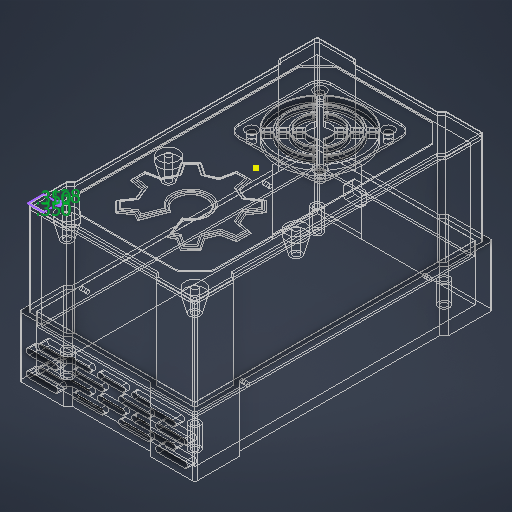
# Autodesk Inventor part: OSHE_ClassH_Enclosure_v2.0
Saved by Autodesk Inventor 2026.2 (Build 302298000, 298)
## iProperties
Created: 2026-04-01
Part Number: OSHE_ClassH_Enclosure_v2.0
Material: Generic
Document SubType Name: Modeling
Designer: ODFab
Density: 1 g/cm^3
Appearance: Default
Author: ODFab
Autodesk Inventor part; units mm, degrees
(part 1 of 2)
ref_plane "YZ Plane" through (0, 0, 0) normal (1, 0, 0) x (0, 1, 0)
ref_plane "XZ Plane" through (0, 0, 0) normal (0, 1, 0) x (-1, 0, 0)
ref_plane "XY Plane" through (0, 0, 0) normal (0, 0, 1) x (1, 0, 0)
sketch "Sketch1" plane through (0, 0, 0) normal (0, 1, 0) x (-1, 0, 0)
  line L0 (41.275, 76.2) -> (-41.275, 76.2)
  line L1 (-41.275, 76.2) -> (-41.275, -76.2)
  line L2 (-41.275, -76.2) -> (41.275, -76.2)
  line L3 (41.275, -76.2) -> (41.275, 76.2)
  line L4 (41.275, 76.2) -> (-41.275, -76.2) construction
  line L5 (-41.275, 76.2) -> (41.275, -76.2) construction
  line L6 (45.085, 80.01) -> (-45.085, 80.01)
  line L7 (-45.085, 80.01) -> (-45.085, -80.01)
  line L8 (-45.085, -80.01) -> (45.085, -80.01)
  line L9 (45.085, -80.01) -> (45.085, 80.01)
  line L10 (47.625, 82.55) -> (-47.625, 82.55)
  line L11 (-47.625, 82.55) -> (-47.625, -82.55)
  line L12 (-47.625, -82.55) -> (47.625, -82.55)
  line L13 (47.625, -82.55) -> (47.625, 82.55)
  line L14 (50.165, 85.09) -> (-50.165, 85.09)
  line L15 (-50.165, 85.09) -> (-50.165, -85.09)
  line L16 (-50.165, -85.09) -> (50.165, -85.09)
  line L17 (50.165, -85.09) -> (50.165, 85.09)
  line L18 (50.165, -85.09) -> (24.765, -85.09)
  line L19 (24.765, -85.09) -> (24.765, -59.69)
  line L20 (24.765, -59.69) -> (50.165, -59.69)
  line L21 (50.165, -59.69) -> (50.165, -85.09)
  line L22 (50.165, -59.69) -> (47.625, -59.69)
  line L23 (47.625, -59.69) -> (47.625, -57.15)
  line L24 (47.625, -57.15) -> (50.165, -57.15)
  line L25 (50.165, -57.15) -> (50.165, -59.69)
  line L26 (24.765, -82.55) -> (22.225, -82.55)
  line L27 (22.225, -82.55) -> (22.225, -85.09)
  line L28 (22.225, -85.09) -> (24.765, -85.09)
  line L29 (24.765, -85.09) -> (24.765, -82.55)
  line L30 (24.765, -85.09) -> (22.225, -82.55)
  line L31 (50.165, -59.69) -> (47.625, -57.15)
  line L32 (0, -85.09) -> (0, -83.82)
  line L33 (-50.165, 0) -> (-49.2125, 0)
  line L34 (-24.765, -85.09) -> (-22.225, -82.55)
  line L35 (-50.165, -59.69) -> (-47.625, -57.15)
  line L36 (24.765, 85.09) -> (22.225, 82.55)
  line L37 (50.165, 59.69) -> (47.625, 57.15)
  line L38 (-24.765, 85.09) -> (-22.225, 82.55)
  line L39 (-50.165, 59.69) -> (-47.625, 57.15)
  point P0 (0, 0)
  dimension "d0" = 82.55
  dimension "d1" = 152.4
  dimension "d2" = 3.81
  dimension "d3" = 2.54
  dimension "d4" = 2.54
  dimension "d5" = 25.4
  dimension "d6" = 25.4
  dimension "d7" = 2.54
  dimension "d8" = 2.54
  dimension "d9" = 2.54
  dimension "d10" = 2.54
  constraints: 80 end point, 14 parallel, 12 symmetric about line, 7 perpendicular, 5 horizontal, 4 midpoint, 2 point on line, 1 vertical, 9 other
  measures "d0" distance of L2.end L1.end
  measures "d1" distance of L1.end L0.end
  measures "d2" distance between parallel lines of L3 L9
  measures "d3" distance between parallel lines of L9 L13
  measures "d4" distance between parallel lines of L13 L17
  measures "d5" distance of L19.end L20.end
  measures "d6" distance of L18.end L19.end
  measures "d7" distance of L23.end L24.end
  measures "d8" distance of L22.end L23.end
  measures "d9" distance of L28.end L27.end
  measures "d10" distance of L27.end L26.end
extrude "Extrusion1" add sketch "Sketch1" along normal blind 31.75 contours L20 L13 L12 L19 L8 L9 | L9 L6 L7 L8 L19 L12 L11 L10 L13 L20 | L20 L17 L16 L19 L12 L13 | L13 L31 L20 | L19 L30 L12 | L13 L10 L36 L14 L17 L37 | L34 L16 L15 L35 L11 L12 | L10 L11 L39 L15 L14 L38
ref_plane "Work Plane1" through (-50.165, 0, 59.69) normal (-1, 0, 0) x (0, 0, 1)
sketch "Sketch2" plane through (-50.165, 0, 59.69) normal (-1, 0, 0) x (0, 0, 1)
  line L0 (-144.78, 0) -> (-119.38, 0) projected
  line L1 (-119.38, 0) -> (-119.38, 31.75) projected
  line L2 (-144.78, 31.75) -> (-119.38, 31.75) projected
  line L3 (-144.78, 0) -> (-144.78, 31.75) projected
  line L4 (0, 0) -> (25.4, 0) projected
  line L5 (25.4, 0) -> (25.4, 31.75) projected
  line L6 (0, 31.75) -> (25.4, 31.75) projected
  line L7 (0, 0) -> (0, 31.75) projected
  line L8 (-144.78, 31.75) -> (25.4, 31.75)
  line L9 (25.4, 31.75) -> (25.4, 0)
  line L10 (25.4, 0) -> (-144.78, 0)
  line L11 (-144.78, 0) -> (-144.78, 31.75)
  line L12 (-144.78, 0) -> (25.4, 0)
  line L13 (25.4, 0) -> (25.4, -2.54)
  line L14 (25.4, -2.54) -> (-144.78, -2.54)
  line L15 (-144.78, -2.54) -> (-144.78, 0)
  point P0 (-59.69, 0)
  point P1 (-119.38, 0)
  dimension "d14" = 2.54
  constraints: 16 end point, 4 parallel, 2 horizontal, 2 perpendicular, 1 point on line
  measures "d14" distance of L12.end L13.end
extrude "Extrusion2" add sketch "Sketch2" against normal up to surface (100.33 mm away) contours L0 L10 L4 L13 L14 L15
sketch "Sketch3" plane through (0, 31.75, 0) normal (0, 1, 0) x (1, 0, 0)
  line L0 (-47.625, 57.15) -> (-47.625, -57.15) projected
  line L1 (-47.625, -57.15) -> (-50.165, -59.69) projected
  line L2 (-50.165, -59.69) -> (-50.165, -85.09) projected
  line L3 (-50.165, -85.09) -> (-24.765, -85.09) projected
  line L4 (-24.765, -85.09) -> (-22.225, -82.55) projected
  line L5 (-22.225, -82.55) -> (22.225, -82.55) projected
  line L6 (22.225, -82.55) -> (24.765, -85.09) projected
  line L7 (24.765, -85.09) -> (50.165, -85.09) projected
  line L8 (50.165, -85.09) -> (50.165, -59.69) projected
  line L9 (50.165, -59.69) -> (47.625, -57.15) projected
  line L10 (47.625, -57.15) -> (47.625, 57.15) projected
  line L11 (47.625, 57.15) -> (50.165, 59.69) projected
  line L12 (50.165, 59.69) -> (50.165, 85.09) projected
  line L13 (50.165, 85.09) -> (24.765, 85.09) projected
  line L14 (24.765, 85.09) -> (22.225, 82.55) projected
  line L15 (22.225, 82.55) -> (-22.225, 82.55) projected
  line L16 (-22.225, 82.55) -> (-24.765, 85.09) projected
  line L17 (-24.765, 85.09) -> (-50.165, 85.09) projected
  line L18 (-50.165, 85.09) -> (-50.165, 59.69) projected
  line L19 (-50.165, 59.69) -> (-47.625, 57.15) projected
  line L20 (-45.085, 80.01) -> (45.085, 80.01) projected
  line L21 (45.085, 80.01) -> (45.085, -80.01) projected
  line L22 (45.085, -80.01) -> (-45.085, -80.01) projected
  line L23 (-45.085, -80.01) -> (-45.085, 80.01) projected
  line L24 (-50.165, 85.09) -> (50.165, 85.09)
  line L25 (50.165, 85.09) -> (50.165, -85.09)
  line L26 (50.165, -85.09) -> (-50.165, -85.09)
  line L27 (-50.165, -85.09) -> (-50.165, 85.09)
  point P0 (0, 0)
  constraints: 8 end point, 2 parallel, 1 horizontal, 1 perpendicular
extrude "Extrusion3" cut sketch "Sketch3" against normal up to surface (34.29 mm away) contours L0 L1 L27 L19 | L24 L14 L15 L16 | L4 L5 L6 L26 | L25 L9 L10 L11
sketch "Sketch4" plane through (-45.085, 0, 80.01) normal (0, 1, 0) x (1, 0, 0)
  line L0 (86.36, 3.81) -> (3.81, 3.81)
  line L1 (3.81, 3.81) -> (3.81, 156.21)
  line L2 (3.81, 156.21) -> (86.36, 156.21)
  line L3 (86.36, 156.21) -> (86.36, 3.81)
  line L4 (86.36, 3.81) -> (3.81, 156.21) construction
  line L5 (3.81, 3.81) -> (86.36, 156.21) construction
  line L6 (3.81, 156.21) -> (8.89, 156.21)
  line L7 (8.89, 156.21) -> (8.89, 151.13)
  line L8 (8.89, 151.13) -> (3.81, 151.13)
  line L9 (3.81, 151.13) -> (3.81, 156.21)
  circle A0 centre (8.89, 151.13) radius 1.7526
  line L10 (45.085, 156.21) -> (45.085, 155.0838)
  line L11 (86.36, 80.01) -> (84.9425, 80.01)
  circle A1 centre (8.89, 151.13) radius 3.0226
  circle A2 centre (81.28, 151.13) radius 1.7526
  circle A3 centre (81.28, 151.13) radius 3.0226
  circle A4 centre (8.89, 8.89) radius 1.7526
  circle A5 centre (8.89, 8.89) radius 3.0226
  circle A6 centre (81.28, 8.89) radius 3.0226
  circle A7 centre (81.28, 8.89) radius 1.7526
  point P0 (45.085, 80.01)
  dimension "d19" = 82.55
  dimension "d20" = 152.4
  dimension "d21" = 5.08
  dimension "d22" = 5.08
  dimension "d23" = 3.5052
  dimension "d24" = 1.27
  constraints: 24 end point, 8 centre point, 4 midpoint, 4 parallel, 3 horizontal, 3 symmetric about line, 2 perpendicular, 1 coincident, 1 vertical, 6 other
  measures "d19" distance of L1.end L2.end
  measures "d20" distance of L0.end L1.end
  measures "d21" distance of L7.end L8.end
  measures "d22" distance of L6.end L7.end
  measures "d23" diameter of A0
  measures "d24" radial gap between concentric circles of A0 A1
extrude "Extrusion4" add sketch "Sketch4" along normal blind 12.7 contours A1 L7 A0 L8 | L8 A0 L7 A1 | A3 | A5 | A6
fillet "Fillet1" radius 1.27 7 edges at (-50.165, 14.605, -85.09) (50.165, 15.875, -85.09) (50.165, -1.27, -85.09) (50.165, 15.875, 85.09) (50.165, -1.27, 85.09) (-50.165, 15.875, 85.09) (-50.165, -1.27, 85.09)
sketch "Sketch5" plane through (-24.765, -2.54, -85.09) normal (0, 0, -1) x (-1, 0, 0)
  line L0 (24.13, 34.29) -> (24.13, 0) projected
  line L1 (0, 34.29) -> (24.13, 34.29) projected
  line L2 (0, 0) -> (0, 34.29) projected
  line L3 (24.13, 0) -> (0, 0) projected
  line L4 (20.32, 2.54) -> (20.32, 34.29) projected
  line L5 (20.32, 21.4335) -> (5.08, 21.4335)
  line L6 (5.08, 21.4335) -> (-5.0723, 21.4335)
  line L7 (-5.0723, 21.4335) -> (-5.0723, 23.9735)
  line L8 (-5.0723, 21.4335) -> (-5.0723, 17.6235)
  line L9 (-3.8023, 25.2435) -> (3.81, 25.2435)
  line L10 (5.08, 23.9735) -> (5.08, 18.8935)
  line L11 (3.81, 17.6235) -> (-3.8023, 17.6235)
  line L12 (-5.0723, 18.8935) -> (-5.0723, 25.2435)
  arc A0 (-3.8023, 25.2435) -> (-5.0723, 23.9735) centre (-3.8023, 23.9735) ccw
  arc A1 (5.08, 23.9735) -> (3.81, 25.2435) centre (3.81, 23.9735) ccw
  arc A2 (-5.0723, 18.8935) -> (-3.8023, 17.6235) centre (-3.8023, 18.8935) ccw
  arc A3 (3.81, 17.6235) -> (5.08, 18.8935) centre (3.81, 18.8935) ccw
  point P0 (-24.765, 2.54)
  dimension "d28" = 15.24
  dimension "d29" = 3.81
  dimension "d30" = 3.81
  dimension "d31" = 1.27
  constraints: 16 end point, 8 point on circle, 8 tangent, 4 centre point, 3 equal radius, 3 horizontal, 3 point on line, 2 parallel, 2 vertical, 1 perpendicular
  measures "d28" distance of L5.start L5.end
  measures "d29" distance of L6.end L12.end
  measures "d30" distance of L6.end L8.end
  measures "d31" radius of A0
extrude "Extrusion5" cut sketch "Sketch5" against normal blind 31.75 contours L11 A2 L8 L6 L2 | L2 L6 L10 A3 L11 | L9 A1 L10 L6 L2 | L2 L6 L7 A0 L9
sketch "Sketch6" plane through (24.765, -2.54, 85.09) normal (0, 0, 1) x (1, 0, 0)
  line L0 (-73.66, 0) -> (-73.66, 34.29) projected
  line L1 (-73.66, 0) -> (-49.53, 0) projected
  line L2 (-49.53, 0) -> (-49.53, 34.29) projected
  line L3 (-73.66, 34.29) -> (-49.53, 34.29) projected
  line L4 (24.13, 34.29) -> (24.13, 0) projected
  line L5 (0, 34.29) -> (24.13, 34.29) projected
  line L6 (0, 0) -> (0, 34.29) projected
  line L7 (0, 0) -> (24.13, 0) projected
  line L8 (25.4, 0) -> (25.4, 34.29) projected
  line L9 (-74.93, 34.29) -> (-74.93, 0) projected
  line L10 (-74.93, 34.29) -> (-73.66, 34.29) projected
  line L11 (-73.66, 0) -> (-74.93, 0) projected
  line L12 (24.13, 34.29) -> (25.4, 34.29) projected
  line L13 (25.4, 0) -> (24.13, 0) projected
  line L14 (-74.93, 34.29) -> (25.4, 34.29)
  line L15 (25.4, 34.29) -> (25.4, 0)
  line L16 (25.4, 0) -> (-74.93, 0)
  line L17 (-74.93, 0) -> (-74.93, 34.29)
  line L18 (-2.54, 34.29) -> (-46.99, 34.29) projected
  line L19 (-74.93, 0) -> (-24.765, 0)
  line L20 (-24.765, 0) -> (-24.765, 34.29)
  line L21 (-24.765, 34.29) -> (-74.93, 34.29)
  line L22 (-74.93, 34.29) -> (-74.93, 0)
  line L23 (-74.93, 34.29) -> (-24.765, 34.29)
  line L24 (-49.8475, 22.86) -> (-49.8475, 0)
  line L25 (-73.66, 0) -> (-49.53, 0) projected
  line L26 (-74.93, 34.29) -> (-74.93, 22.86)
  line L27 (-74.93, 22.86) -> (-74.93, 11.43)
  line L28 (-74.93, 0) -> (-74.93, 34.29) projected
  line L29 (-74.93, 11.43) -> (-74.93, 0)
  line L30 (-74.93, 22.86) -> (-49.8475, 22.86)
  line L31 (-74.93, 11.43) -> (-49.8475, 11.43)
  line L32 (-73.66, 22.86) -> (-69.215, 22.86)
  line L33 (-69.215, 22.86) -> (-69.215, 28.575)
  line L34 (-69.215, 28.575) -> (-73.66, 28.575)
  line L35 (-73.66, 28.575) -> (-73.66, 22.86)
  arc A0 (-69.215, 30.2385) -> (-69.215, 26.9115) centre (-69.215, 28.575) ccw
  line L36 (-74.93, 34.29) -> (25.4, 34.29)
  line L37 (25.4, 34.29) -> (25.4, 36.83)
  line L38 (25.4, 36.83) -> (-74.93, 36.83)
  line L39 (-74.93, 36.83) -> (-74.93, 34.29)
  line L40 (-74.93, 36.83) -> (-24.765, 36.83)
  line L41 (-24.765, 36.83) -> (-24.765, 40.0775)
  line L42 (-24.765, 40.0775) -> (-74.93, 40.0775)
  line L43 (-74.93, 40.0775) -> (-74.93, 36.83)
  line L44 (-49.8475, 22.86) -> (-54.2925, 22.86)
  line L45 (-54.2925, 22.86) -> (-54.2925, 28.575)
  line L46 (-54.2925, 28.575) -> (-49.8475, 28.575)
  line L47 (-49.8475, 28.575) -> (-49.8475, 22.86)
  arc A1 (-54.2925, 26.9115) -> (-54.2925, 30.2385) centre (-54.2925, 28.575) ccw
  line L48 (-69.215, 30.2385) -> (-54.2925, 30.2385)
  line L49 (-69.215, 26.9115) -> (-54.2925, 26.9115)
  arc A2 (-69.215, 18.8085) -> (-69.215, 15.4815) centre (-69.215, 17.145) ccw
  arc A3 (-54.2925, 15.4815) -> (-54.2925, 18.8085) centre (-54.2925, 17.145) ccw
  line L50 (-69.215, 15.4815) -> (-54.2925, 15.4815)
  line L51 (-69.215, 18.8085) -> (-54.2925, 18.8085)
  arc A4 (-69.215, 7.3785) -> (-69.215, 4.0515) centre (-69.215, 5.715) ccw
  line L52 (-69.215, 7.3785) -> (-54.2925, 7.3785)
  line L53 (-69.215, 4.0515) -> (-54.2925, 4.0515)
  arc A5 (-54.2925, 4.0515) -> (-54.2925, 7.3785) centre (-54.2925, 5.715) ccw
  arc A6 (-30.48, 26.9115) -> (-30.48, 30.2385) centre (-30.48, 28.575) ccw
  arc A7 (-45.4025, 30.2385) -> (-45.4025, 26.9115) centre (-45.4025, 28.575) ccw
  line L54 (-30.48, 30.2385) -> (-45.4025, 30.2385)
  line L55 (-30.48, 26.9115) -> (-45.4025, 26.9115)
  arc A8 (-62.3887, 24.5235) -> (-62.3887, 21.1965) centre (-62.3887, 22.86) ccw
  line L56 (-45.4025, 28.575) -> (-30.48, 28.575)
  arc A9 (-37.9412, 21.1965) -> (-37.9412, 24.5235) centre (-37.9412, 22.86) ccw
  line L57 (-62.3887, 24.5235) -> (-37.9412, 24.5235)
  line L58 (-37.9412, 21.1965) -> (-62.3887, 21.1965)
  arc A10 (-30.48, 15.4815) -> (-30.48, 18.8085) centre (-30.48, 17.145) ccw
  line L59 (-30.48, 15.4815) -> (-45.4025, 15.4815)
  line L60 (-30.48, 18.8085) -> (-45.4025, 18.8085)
  arc A11 (-45.4025, 18.8085) -> (-45.4025, 15.4815) centre (-45.4025, 17.145) ccw
  line L61 (-30.48, 4.0515) -> (-45.4025, 4.0515)
  arc A12 (-30.48, 4.0515) -> (-30.48, 7.3785) centre (-30.48, 5.715) ccw
  line L62 (-30.48, 7.3785) -> (-45.4025, 7.3785)
  arc A13 (-45.4025, 7.3785) -> (-45.4025, 4.0515) centre (-45.4025, 5.715) ccw
  line L63 (-54.2925, 17.145) -> (-53.9161, 17.145)
  arc A14 (-62.3887, 13.0935) -> (-62.3887, 9.7665) centre (-62.3887, 11.43) ccw
  arc A15 (-37.9412, 9.7665) -> (-37.9412, 13.0935) centre (-37.9412, 11.43) ccw
  line L64 (-62.3887, 9.7665) -> (-37.9412, 9.7665)
  line L65 (-37.9412, 13.0935) -> (-62.3887, 13.0935)
  line L66 (19.685, 22.86) -> (19.685, 28.575)
  arc A16 (19.685, 26.9115) -> (19.685, 30.2385) centre (19.685, 28.575) ccw
  line L67 (0.3175, 22.86) -> (4.7625, 22.86)
  line L68 (4.7625, 22.86) -> (4.7625, 28.575)
  line L69 (4.7625, 28.575) -> (0.3175, 28.575)
  line L70 (0.3175, 28.575) -> (0.3175, 22.86)
  arc A17 (4.7625, 30.2385) -> (4.7625, 26.9115) centre (4.7625, 28.575) ccw
  line L71 (19.685, 30.2385) -> (4.7625, 30.2385)
  line L72 (19.685, 26.9115) -> (4.7625, 26.9115)
  arc A18 (19.685, 15.4815) -> (19.685, 18.8085) centre (19.685, 17.145) ccw
  line L73 (19.685, 15.4815) -> (4.7625, 15.4815)
  line L74 (19.685, 18.8085) -> (4.7625, 18.8085)
  arc A19 (4.7625, 18.8085) -> (4.7625, 15.4815) centre (4.7625, 17.145) ccw
  line L75 (19.685, 4.0515) -> (4.7625, 4.0515)
  arc A20 (19.685, 4.0515) -> (19.685, 7.3785) centre (19.685, 5.715) ccw
  line L76 (19.685, 7.3785) -> (4.7625, 7.3785)
  arc A21 (4.7625, 7.3785) -> (4.7625, 4.0515) centre (4.7625, 5.715) ccw
  line L77 (-19.05, 30.2385) -> (-4.1275, 30.2385)
  arc A22 (-19.05, 30.2385) -> (-19.05, 26.9115) centre (-19.05, 28.575) ccw
  line L78 (-19.05, 26.9115) -> (-4.1275, 26.9115)
  arc A23 (-4.1275, 26.9115) -> (-4.1275, 30.2385) centre (-4.1275, 28.575) ccw
  arc A24 (12.8588, 21.1965) -> (12.8588, 24.5235) centre (12.8588, 22.86) ccw
  line L79 (-4.1275, 28.575) -> (-19.05, 28.575)
  arc A25 (-11.5887, 24.5235) -> (-11.5887, 21.1965) centre (-11.5887, 22.86) ccw
  line L80 (12.8588, 24.5235) -> (-11.5887, 24.5235)
  line L81 (-11.5887, 21.1965) -> (12.8588, 21.1965)
  line L82 (-19.05, 18.8085) -> (-4.1275, 18.8085)
  arc A26 (-19.05, 18.8085) -> (-19.05, 15.4815) centre (-19.05, 17.145) ccw
  line L83 (-19.05, 15.4815) -> (-4.1275, 15.4815)
  arc A27 (-4.1275, 15.4815) -> (-4.1275, 18.8085) centre (-4.1275, 17.145) ccw
  line L84 (-19.05, 7.3785) -> (-4.1275, 7.3785)
  arc A28 (-4.1275, 4.0515) -> (-4.1275, 7.3785) centre (-4.1275, 5.715) ccw
  line L85 (-19.05, 4.0515) -> (-4.1275, 4.0515)
  arc A29 (-19.05, 7.3785) -> (-19.05, 4.0515) centre (-19.05, 5.715) ccw
  line L86 (4.7625, 17.145) -> (4.3861, 17.145)
  line L87 (12.8588, 9.7665) -> (-11.5887, 9.7665)
  arc A30 (12.8588, 9.7665) -> (12.8588, 13.0935) centre (12.8588, 11.43) ccw
  line L88 (-11.5887, 13.0935) -> (12.8588, 13.0935)
  arc A31 (-11.5887, 13.0935) -> (-11.5887, 9.7665) centre (-11.5887, 11.43) ccw
  arc A32 (-31.0475, 24.5235) -> (-31.0475, 21.1965) centre (-31.0475, 22.86) ccw
  line L89 (-31.0475, 24.5235) -> (-24.765, 24.5235)
  line L90 (-31.0475, 21.1965) -> (-24.765, 21.1965)
  arc A33 (-18.4825, 21.1965) -> (-18.4825, 24.5235) centre (-18.4825, 22.86) ccw
  line L91 (-18.4825, 24.5235) -> (-24.765, 24.5235)
  line L92 (-18.4825, 21.1965) -> (-24.765, 21.1965)
  arc A34 (-31.0475, 13.0935) -> (-31.0475, 9.7665) centre (-31.0475, 11.43) ccw
  line L93 (-31.0475, 9.7665) -> (-24.765, 9.7665)
  line L94 (-31.0475, 13.0935) -> (-24.765, 13.0935)
  line L95 (-18.4825, 9.7665) -> (-24.765, 9.7665)
  arc A35 (-18.4825, 9.7665) -> (-18.4825, 13.0935) centre (-18.4825, 11.43) ccw
  line L96 (-18.4825, 13.0935) -> (-24.765, 13.0935)
  point P0 (-24.765, 2.54)
  point P1 (0.3175, 11.43)
  point P2 (-49.53, 13.0935)
  point P3 (-49.53, 21.1965)
  point P4 (-49.8475, 21.1965)
  point P5 (-49.8475, 13.0935)
  point P6 (3.099, 28.575)
  dimension "d34" = 11.43
  dimension "d35" = 11.43
  dimension "d36" = 4.445
  dimension "d37" = 5.715
  dimension "d38" = 3.327
  dimension "d40" = 2.54
  dimension "d41" = 4.445
  dimension "d42" = 5.715
  dimension "d43" = 3.327
  dimension "d44" = 3.327
  dimension "d45" = 3.327
  dimension "d46" = 3.327
  constraints: 160 end point, 103 symmetric about line, 72 point on circle, 36 centre point, 12 parallel, 12 point on line, 11 perpendicular, 7 horizontal, 5 tangent, 4 coincident, 3 midpoint, 2 collinear, 31 other
  measures "d34" distance of L21.end L26.end
  measures "d35" distance of L26.end L27.end
  measures "d36" distance of L34.end L33.end
  measures "d37" distance of L33.end L32.end
  measures "d38" diameter of A0
  measures "d40" distance of L37.end L36.end
  measures "d41" distance of L45.end L46.end
  measures "d42" distance of L44.end L45.end
  measures "d43" diameter of A1
  measures "d44" diameter of A8
  measures "d45" diameter of A9
  measures "d46" diameter of A32
extrude "Extrusion6" cut sketch "Sketch6" against normal up to surface (5.08 mm away) contours A14 L65 L24 L31 | L31 L24 L64 A14 | A8 L57 L45 L30 | L30 L24 L58 A8 | L24 L65 L2 L64 | L45 L57 L47 L30 | L57 A9 L58 L2 | L2 L58 L24 L47 L57 | L2 L65 A15 L64 | L91 A33 L92 L20 | L20 L90 A32 L89 | L93 A34 L94 L20 | L20 L96 A35 L95 | L87 A31 L88 L6 | L6 L88 A30 L87 | L80 L70 L67 L68 A24 L81 L6 | L6 L81 A25 L80 | L80 L68 L67 L70 | L51 A3 L50 A2 | L52 A5 L53 A4 | L59 A11 L60 A10 | L61 A13 L62 A12 | L73 A19 L74 A18 | L75 A21 L76 A20 | L82 A27 L83 A26 | L84 A28 L85 A29
ref_plane "Work Plane2" through (0, 31.75, 0) normal (0, 1, 0) x (1, 0, 0)
sketch "Sketch7" plane through (0, 31.75, 0) normal (0, 1, 0) x (1, 0, 0)
  arc A0 (-50.165, -83.82) -> (-48.895, -85.09) centre (-48.895, -83.82) ccw projected
  line L0 (-48.895, -85.09) -> (-24.765, -85.09) projected
  line L1 (-24.765, -85.09) -> (-22.225, -82.55) projected
  line L2 (-22.225, -82.55) -> (22.225, -82.55) projected
  line L3 (22.225, -82.55) -> (24.765, -85.09) projected
  line L4 (24.765, -85.09) -> (48.895, -85.09) projected
  arc A1 (48.895, -85.09) -> (50.165, -83.82) centre (48.895, -83.82) ccw projected
  line L5 (50.165, -83.82) -> (50.165, -59.69) projected
  line L6 (50.165, -59.69) -> (47.625, -57.15) projected
  line L7 (47.625, -57.15) -> (47.625, 57.15) projected
  line L8 (47.625, 57.15) -> (50.165, 59.69) projected
  line L9 (50.165, 59.69) -> (50.165, 83.82) projected
  arc A2 (50.165, 83.82) -> (48.895, 85.09) centre (48.895, 83.82) ccw projected
  line L10 (48.895, 85.09) -> (24.765, 85.09) projected
  line L11 (24.765, 85.09) -> (22.225, 82.55) projected
  line L12 (22.225, 82.55) -> (-22.225, 82.55) projected
  line L13 (-22.225, 82.55) -> (-24.765, 85.09) projected
  line L14 (-24.765, 85.09) -> (-48.895, 85.09) projected
  arc A3 (-48.895, 85.09) -> (-50.165, 83.82) centre (-48.895, 83.82) ccw projected
  line L15 (-50.165, 83.82) -> (-50.165, 59.69) projected
  line L16 (-50.165, 59.69) -> (-47.625, 57.15) projected
  line L17 (-47.625, 57.15) -> (-47.625, -57.15) projected
  line L18 (-47.625, -57.15) -> (-50.165, -59.69) projected
  line L19 (-50.165, -59.69) -> (-50.165, -83.82) projected
  line L20 (-45.085, 80.01) -> (45.085, 80.01) projected
  line L21 (45.085, 80.01) -> (45.085, -80.01) projected
  line L22 (45.085, -80.01) -> (-45.085, -80.01) projected
  line L23 (-45.085, -80.01) -> (-45.085, 80.01) projected
  circle A4 centre (-36.195, -71.12) radius 3.0226 projected
  circle A5 centre (36.195, 71.12) radius 3.0226 projected
  circle A6 centre (36.195, -71.12) radius 3.0226 projected
  circle A7 centre (-36.195, 71.12) radius 3.0226 projected
  line L24 (-45.085, -80.01) -> (-45.085, 80.01) projected
  line L25 (45.085, -80.01) -> (-45.085, -80.01) projected
  line L26 (45.085, 80.01) -> (45.085, -80.01) projected
  line L27 (-45.085, 80.01) -> (45.085, 80.01) projected
  line L28 (-47.625, 82.55) -> (-25.8171, 82.55)
  line L29 (-25.8171, 82.55) -> (-23.2771, 80.01)
  line L30 (-23.2771, 80.01) -> (23.2771, 80.01)
  line L31 (23.2771, 80.01) -> (25.8171, 82.55)
  line L32 (25.8171, 82.55) -> (47.625, 82.55)
  line L33 (47.625, 82.55) -> (47.625, 60.7421)
  line L34 (47.625, 60.7421) -> (45.085, 58.2021)
  line L35 (45.085, 58.2021) -> (45.085, -58.2021)
  line L36 (45.085, -58.2021) -> (47.625, -60.7421)
  line L37 (47.625, -60.7421) -> (47.625, -82.55)
  line L38 (47.625, -82.55) -> (25.8171, -82.55)
  line L39 (25.8171, -82.55) -> (23.2771, -80.01)
  line L40 (23.2771, -80.01) -> (-23.2771, -80.01)
  line L41 (-23.2771, -80.01) -> (-25.8171, -82.55)
  line L42 (-25.8171, -82.55) -> (-47.625, -82.55)
  line L43 (-47.625, -82.55) -> (-47.625, -60.7421)
  line L44 (-47.625, -60.7421) -> (-45.085, -58.2021)
  line L45 (-45.085, -58.2021) -> (-45.085, 58.2021)
  line L46 (-45.085, 58.2021) -> (-47.625, 60.7421)
  line L47 (-47.625, 60.7421) -> (-47.625, 82.55)
  line L48 (-44.985, 79.91) -> (44.985, 79.91)
  line L49 (44.985, 79.91) -> (44.985, -79.91)
  line L50 (44.985, -79.91) -> (-44.985, -79.91)
  line L51 (-44.985, -79.91) -> (-44.985, 79.91)
  line L52 (-43.715, 78.64) -> (43.715, 78.64)
  line L53 (43.715, 78.64) -> (43.715, -78.64)
  line L54 (43.715, -78.64) -> (-43.715, -78.64)
  line L55 (-43.715, -78.64) -> (-43.715, 78.64)
  point P0 (0, 0)
  dimension "d50" = 2.54
  dimension "d51" = 0.1
  dimension "d52" = 1.27
  constraints: 56 end point, 25 other
  measures "d50" distance between parallel lines of L14 L28
  measures "d51" distance between parallel lines of L23 L51
  measures "d52" distance between parallel lines of L51 L55
extrude "Extrusion7" add sketch "Sketch7" against normal blind 7.62 separate body contours L48 L49 L50 L51
sketch "Sketch8" plane through (0, 31.75, 0) normal (0, 1, 0) x (1, 0, 0)
  line L0 (-44.985, -79.91) -> (44.985, -79.91) projected
  line L1 (44.985, -79.91) -> (44.985, 79.91) projected
  line L2 (44.985, 79.91) -> (-44.985, 79.91) projected
  line L3 (-44.985, 79.91) -> (-44.985, -79.91) projected
  line L4 (-43.715, 78.64) -> (43.715, 78.64) projected
  line L5 (43.715, 78.64) -> (43.715, -78.64) projected
  line L6 (43.715, -78.64) -> (-43.715, -78.64) projected
  line L7 (-43.715, -78.64) -> (-43.715, 78.64) projected
  arc A0 (-50.165, -83.82) -> (-48.895, -85.09) centre (-48.895, -83.82) ccw projected
  line L8 (-48.895, -85.09) -> (-24.765, -85.09) projected
  line L9 (-24.765, -85.09) -> (-22.225, -82.55) projected
  line L10 (-22.225, -82.55) -> (22.225, -82.55) projected
  line L11 (22.225, -82.55) -> (24.765, -85.09) projected
  line L12 (24.765, -85.09) -> (48.895, -85.09) projected
  arc A1 (48.895, -85.09) -> (50.165, -83.82) centre (48.895, -83.82) ccw projected
  line L13 (50.165, -83.82) -> (50.165, -59.69) projected
  line L14 (50.165, -59.69) -> (47.625, -57.15) projected
  line L15 (47.625, -57.15) -> (47.625, 57.15) projected
  line L16 (47.625, 57.15) -> (50.165, 59.69) projected
  line L17 (50.165, 59.69) -> (50.165, 83.82) projected
  arc A2 (50.165, 83.82) -> (48.895, 85.09) centre (48.895, 83.82) ccw projected
  line L18 (48.895, 85.09) -> (24.765, 85.09) projected
  line L19 (24.765, 85.09) -> (22.225, 82.55) projected
  line L20 (22.225, 82.55) -> (-22.225, 82.55) projected
  line L21 (-22.225, 82.55) -> (-24.765, 85.09) projected
  line L22 (-24.765, 85.09) -> (-48.895, 85.09) projected
  arc A3 (-48.895, 85.09) -> (-50.165, 83.82) centre (-48.895, 83.82) ccw projected
  line L23 (-50.165, 83.82) -> (-50.165, 59.69) projected
  line L24 (-50.165, 59.69) -> (-47.625, 57.15) projected
  line L25 (-47.625, 57.15) -> (-47.625, -57.15) projected
  line L26 (-47.625, -57.15) -> (-50.165, -59.69) projected
  line L27 (-50.165, -59.69) -> (-50.165, -83.82) projected
  line L28 (-45.085, 80.01) -> (45.085, 80.01) projected
  line L29 (45.085, 80.01) -> (45.085, -80.01) projected
  line L30 (45.085, -80.01) -> (-45.085, -80.01) projected
  line L31 (-45.085, -80.01) -> (-45.085, 80.01) projected
  line L32 (-47.625, -82.55) -> (-25.8171, -82.55)
  line L33 (-25.8171, -82.55) -> (-23.2771, -80.01)
  line L34 (-23.2771, -80.01) -> (23.2771, -80.01)
  line L35 (23.2771, -80.01) -> (25.8171, -82.55)
  line L36 (25.8171, -82.55) -> (47.625, -82.55)
  line L37 (47.625, -82.55) -> (47.625, -60.7421)
  line L38 (47.625, -60.7421) -> (45.085, -58.2021)
  line L39 (45.085, -58.2021) -> (45.085, 58.2021)
  line L40 (45.085, 58.2021) -> (47.625, 60.7421)
  line L41 (47.625, 60.7421) -> (47.625, 82.55)
  line L42 (47.625, 82.55) -> (25.8171, 82.55)
  line L43 (25.8171, 82.55) -> (23.2771, 80.01)
  line L44 (23.2771, 80.01) -> (-23.2771, 80.01)
  line L45 (-23.2771, 80.01) -> (-25.8171, 82.55)
  line L46 (-25.8171, 82.55) -> (-47.625, 82.55)
  line L47 (-47.625, 82.55) -> (-47.625, 60.7421)
  line L48 (-47.625, 60.7421) -> (-45.085, 58.2021)
  line L49 (-45.085, 58.2021) -> (-45.085, -58.2021)
  line L50 (-45.085, -58.2021) -> (-47.625, -60.7421)
  line L51 (-47.625, -60.7421) -> (-47.625, -82.55)
  point P0 (0, 0)
  dimension "d0" = 82.55
  dimension "d1" = 152.4
  dimension "d2" = 3.81
  dimension "d3" = 2.54
  dimension "d4" = 2.54
  dimension "d5" = 25.4
  dimension "d6" = 25.4
  dimension "d7" = 2.54
  dimension "d8" = 2.54
  dimension "d9" = 2.54
  dimension "d10" = 2.54
  dimension "d55" = 2.54
  constraints: 40 end point, 19 other
  measures "d55" distance between parallel lines of L27 L51
extrude "Extrusion8" add sketch "Sketch8" along normal blind 50.8 contours L3 L2 L1 L0 | L31 L48 L47 L46 L45 L28 | L28 L29 L30 L31 | L43 L42 L41 L40 L29 L28 | L31 L30 L33 L32 L51 L50 | L38 L37 L36 L35 L30 L29 bodies 2
fillet "Fillet2" radius 1.27 4 edges at (-47.625, 57.15, 82.55) (47.625, 57.15, 82.55) (47.625, 57.15, -82.55) (-47.625, 57.15, -82.55)
sketch "Sketch9" plane through (0, 82.55, 0) normal (0, 1, 0) x (1, 0, 0)
  arc A0 (-46.355, 82.55) -> (-47.625, 81.28) centre (-46.355, 81.28) ccw projected
  line L0 (-47.625, 81.28) -> (-47.625, 60.7421) projected
  line L1 (-47.625, 60.7421) -> (-45.085, 58.2021) projected
  line L2 (-45.085, 58.2021) -> (-45.085, -58.2021) projected
  line L3 (-45.085, -58.2021) -> (-47.625, -60.7421) projected
  line L4 (-47.625, -60.7421) -> (-47.625, -81.28) projected
  arc A1 (-47.625, -81.28) -> (-46.355, -82.55) centre (-46.355, -81.28) ccw projected
  line L5 (-46.355, -82.55) -> (-25.8171, -82.55) projected
  line L6 (-25.8171, -82.55) -> (-23.2771, -80.01) projected
  line L7 (-23.2771, -80.01) -> (23.2771, -80.01) projected
  line L8 (23.2771, -80.01) -> (25.8171, -82.55) projected
  line L9 (25.8171, -82.55) -> (46.355, -82.55) projected
  arc A2 (46.355, -82.55) -> (47.625, -81.28) centre (46.355, -81.28) ccw projected
  line L10 (47.625, -81.28) -> (47.625, -60.7421) projected
  line L11 (47.625, -60.7421) -> (45.085, -58.2021) projected
  line L12 (45.085, -58.2021) -> (45.085, 58.2021) projected
  line L13 (45.085, 58.2021) -> (47.625, 60.7421) projected
  line L14 (47.625, 60.7421) -> (47.625, 81.28) projected
  arc A3 (47.625, 81.28) -> (46.355, 82.55) centre (46.355, 81.28) ccw projected
  line L15 (46.355, 82.55) -> (25.8171, 82.55) projected
  line L16 (25.8171, 82.55) -> (23.2771, 80.01) projected
  line L17 (23.2771, 80.01) -> (-23.2771, 80.01) projected
  line L18 (-23.2771, 80.01) -> (-25.8171, 82.55) projected
  line L19 (-25.8171, 82.55) -> (-46.355, 82.55) projected
  line L20 (-43.715, 78.64) -> (43.715, 78.64) projected
  line L21 (43.715, 78.64) -> (43.715, -78.64) projected
  line L22 (43.715, -78.64) -> (-43.715, -78.64) projected
  line L23 (-43.715, -78.64) -> (-43.715, 78.64) projected
  point P0 (0, 0)
  dimension "d0" = 82.55
  dimension "d1" = 152.4
  dimension "d2" = 3.81
  dimension "d3" = 2.54
  dimension "d4" = 2.54
  dimension "d5" = 25.4
  dimension "d6" = 25.4
  dimension "d7" = 2.54
  dimension "d8" = 2.54
  dimension "d9" = 2.54
  dimension "d10" = 2.54
extrude "Extrusion9" add sketch "Sketch9" along normal blind 2.54 separate body
sketch "Sketch10" plane through (-43.715, 24.13, -78.64) normal (0, 0, 1) x (1, 0, 0)
  line L0 (0, 58.42) -> (0, 0) projected
  line L1 (87.43, 0) -> (0, 0) projected
  line L2 (87.43, 0) -> (87.43, 58.42) projected
  line L3 (0, 60.96) -> (87.43, 60.96)
  line L4 (87.43, 60.96) -> (87.43, 58.42)
  line L5 (87.43, 58.42) -> (0, 58.42)
  line L6 (0, 58.42) -> (0, 60.96)
  line L7 (0, 58.42) -> (87.43, 58.42) projected
  point P0 (43.715, -24.13)
  dimension "d61" = 2.54
  constraints: 8 end point, 2 parallel, 1 horizontal, 1 perpendicular, 1 point on line
  measures "d61" distance of L3.end L4.end
extrude "Extrusion11" add sketch "Sketch10" along normal up to surface (157.28 mm away) contours L6 L3 L4 L5 bodies 3
fillet "Fillet3" radius 0.762 24 edges at (-47.253, 85.09, 82.178) (-47.625, 85.09, 71.0111) (-36.0861, 85.09, 82.55) (0, 85.09, 80.01) (-24.5471, 85.09, 81.28) (24.5471, 85.09, 81.28) (47.253, 85.09, 82.178) (47.625, 85.09, 71.0111) (36.0861, 85.09, 82.55) (46.355, 85.09, 59.4721) (45.085, 85.09, 0) (-45.085, 85.09, 0) (-46.355, 85.09, 59.4721) (46.355, 85.09, -59.4721) (47.253, 85.09, -82.178) (36.0861, 85.09, -82.55) (47.625, 85.09, -71.0111) (24.5471, 85.09, -81.28) (0, 85.09, -80.01) (-24.5471, 85.09, -81.28) (-47.253, 85.09, -82.178) (-47.625, 85.09, -71.0111) (-36.0861, 85.09, -82.55) (-46.355, 85.09, -59.4721)
sketch "Sketch14" plane through (0, 85.09, 0) normal (0, 1, 0) x (1, 0, 0)
  line L0 (-47.625, -82.55) -> (47.625, -82.55)
  line L1 (47.625, -82.55) -> (47.625, 82.55)
  line L2 (47.625, 82.55) -> (-47.625, 82.55)
  line L3 (-47.625, 82.55) -> (-47.625, -82.55)
  line L4 (-26.8879, -73.025) -> (26.8879, -73.025)
  line L5 (38.1, -61.8129) -> (38.1, 61.8129)
  line L6 (26.8879, 73.025) -> (-26.8879, 73.025)
  line L7 (-38.1, 61.8129) -> (-38.1, -61.8129)
  line L8 (-28.6839, -72.2811) -> (-37.3561, -63.6089)
  line L9 (-28.6839, 72.2811) -> (-37.3561, 63.6089)
  line L10 (37.3561, 63.6089) -> (28.6839, 72.2811)
  line L11 (28.6839, -72.2811) -> (37.3561, -63.6089)
  arc A0 (-38.1, -61.8129) -> (-37.3561, -63.6089) centre (-35.56, -61.8129) ccw
  arc A1 (-28.6839, -72.2811) -> (-26.8879, -73.025) centre (-26.8879, -70.485) ccw
  arc A2 (26.8879, -73.025) -> (28.6839, -72.2811) centre (26.8879, -70.485) ccw
  arc A3 (37.3561, -63.6089) -> (38.1, -61.8129) centre (35.56, -61.8129) ccw
  arc A4 (38.1, 61.8129) -> (37.3561, 63.6089) centre (35.56, 61.8129) ccw
  arc A5 (28.6839, 72.2811) -> (26.8879, 73.025) centre (26.8879, 70.485) ccw
  arc A6 (-26.8879, 73.025) -> (-28.6839, 72.2811) centre (-26.8879, 70.485) ccw
  arc A7 (-37.3561, 63.6089) -> (-38.1, 61.8129) centre (-35.56, 61.8129) ccw
  point P0 (0, 0)
  point P1 (-38.1, -73.025)
  point P2 (38.1, -73.025)
  point P3 (38.1, 73.025)
  point P4 (-38.1, 73.025)
  point P5 (-27.94, -73.025)
  point P6 (-38.1, -62.865)
  point P7 (-27.94, 73.025)
  point P8 (-38.1, 62.865)
  point P9 (38.1, 62.865)
  point P10 (27.94, 73.025)
  point P11 (27.94, -73.025)
  point P12 (38.1, -62.865)
  dimension "d79" = 10.16
  dimension "d80" = 10.16
  dimension "d81" = 10.16
  dimension "d82" = 10.16
  dimension "d83" = 10.16
  dimension "d84" = 10.16
  dimension "d85" = 10.16
  dimension "d86" = 10.16
  dimension "d87" = 2.54
  constraints: 24 end point, 24 point on line, 16 point on circle, 16 tangent, 8 centre point, 7 equal radius, 4 parallel, 2 perpendicular, 1 horizontal, 3 other
  measures "d79" distance of point (-27.94, -73.025) point (-38.1, -73.025)
  measures "d80" distance of point (-38.1, -62.865) point (-38.1, -73.025)
  measures "d81" distance of point (-27.94, 73.025) point (-38.1, 73.025)
  measures "d82" distance of point (-38.1, 62.865) point (-38.1, 73.025)
  measures "d83" distance of point (38.1, 62.865) point (38.1, 73.025)
  measures "d84" distance of point (27.94, 73.025) point (38.1, 73.025)
  measures "d85" distance of point (27.94, -73.025) point (38.1, -73.025)
  measures "d86" distance of point (38.1, -62.865) point (38.1, -73.025)
  measures "d87" radius of A0
extrude "Extrusion13" cut sketch "Sketch14" against normal blind 0.635 contours A1 L8 A0 L7 A7 L9 A6 L6 A5 L10 A4 L5 A3 L11 A2 L4 bodies 3
sketch "Sketch16" plane through (0, 84.455, 0) normal (0, 1, 0) x (1, 0, 0)
  line L0 (-32.2834, -2.0503) -> (32.2749, -2.0503) construction
  line L1 (32.2749, -2.0503) -> (32.2749, -66.6086) construction
  line L2 (32.2749, -66.6086) -> (-32.2834, -66.6086) construction
  line L3 (-32.2834, -66.6086) -> (-32.2834, -2.0503) construction
  line L4 (-38.1, -61.8129) -> (-38.1, 61.8129) projected
  circle A0 centre (-0.0042, -37.2738) radius 8.6714
  circle A1 centre (-0.0042, -37.2738) radius 10.2097
  circle A2 centre (-0.0042, -37.2738) radius 21.3565
  line L5 (-3.1296, -45.3624) -> (-3.6841, -46.7973)
  line L6 (-3.6841, -46.7973) -> (-7.7017, -57.1949)
  line L7 (-0.0042, -6.7273) -> (-4.332, -6.7273)
  line L8 (-4.332, -6.7273) -> (-5.999, -15.1705)
  line L9 (-5.999, -15.1705) -> (-11.487, -17.4707)
  line L10 (-11.487, -17.4707) -> (-18.4691, -12.7252)
  line L11 (-18.4691, -12.7252) -> (-24.3757, -18.5553)
  line L12 (-24.3757, -18.5553) -> (-19.6235, -25.496)
  line L13 (-19.6235, -25.496) -> (-22.2149, -31.4918)
  line L14 (-22.2149, -31.4918) -> (-30.3259, -33.0457)
  line L15 (-30.3259, -33.0457) -> (-30.3259, -41.3184)
  line L16 (-30.3259, -41.3184) -> (-22.2893, -42.8055)
  line L17 (-22.2893, -42.8055) -> (-19.7505, -49.0419)
  line L18 (-19.7505, -49.0419) -> (-24.2944, -55.7274)
  line L19 (-24.2944, -55.7274) -> (-18.4691, -61.629)
  line L20 (-18.4691, -61.629) -> (-11.9929, -57.1949)
  line L21 (-11.9929, -57.1949) -> (-8.8207, -58.833)
  line L22 (-8.8207, -58.833) -> (-8.4155, -59.0423)
  line L23 (-8.4155, -59.0423) -> (-7.7017, -57.1949)
  line L24 (-0.0042, -6.7273) -> (-0.0042, -15.9174)
  line L25 (3.6756, -46.7973) -> (7.6932, -57.1949)
  line L26 (-0.0042, -6.7273) -> (4.3235, -6.7273)
  line L27 (4.3235, -6.7273) -> (5.9905, -15.1705)
  line L28 (5.9905, -15.1705) -> (11.4785, -17.4707)
  line L29 (11.4785, -17.4707) -> (18.4606, -12.7252)
  line L30 (18.4606, -12.7252) -> (24.3672, -18.5553)
  line L31 (24.3672, -18.5553) -> (19.615, -25.496)
  line L32 (19.615, -25.496) -> (22.2065, -31.4918)
  line L33 (30.3174, -33.0457) -> (30.3174, -41.3184)
  line L34 (30.3174, -41.3184) -> (22.2808, -42.8055)
  line L35 (22.2808, -42.8055) -> (19.742, -49.0419)
  line L36 (19.742, -49.0419) -> (24.2859, -55.7274)
  line L37 (24.2859, -55.7274) -> (18.4606, -61.629)
  line L38 (18.4606, -61.629) -> (11.9845, -57.1949)
  line L39 (11.9845, -57.1949) -> (8.8123, -58.833)
  line L40 (8.8123, -58.833) -> (8.407, -59.0423)
  line L41 (8.407, -59.0423) -> (7.6932, -57.1949)
  line L42 (22.2065, -31.4918) -> (30.3174, -33.0457)
  line L43 (-7.7092, -57.6746) -> (-11.4012, -55.7681)
  line L44 (-11.4012, -55.7681) -> (-12.1038, -55.4053)
  line L45 (-12.1038, -55.4053) -> (-18.2773, -59.6322)
  line L46 (-18.2773, -59.6322) -> (-22.3102, -55.5464)
  line L47 (-22.3102, -55.5464) -> (-18.014, -49.2252)
  line L48 (-18.014, -49.2252) -> (-21.1811, -41.4452)
  line L49 (-21.1811, -41.4452) -> (-28.7866, -40.0379)
  line L50 (-28.7866, -40.0379) -> (-28.7866, -34.318)
  line L51 (-28.7866, -34.318) -> (-21.1252, -32.8503)
  line L52 (-21.1252, -32.8503) -> (-17.8736, -25.3271)
  line L53 (-17.8736, -25.3271) -> (-22.3788, -18.7471)
  line L54 (-22.3788, -18.7471) -> (-18.2881, -14.7094)
  line L55 (-18.2881, -14.7094) -> (-11.6619, -19.2129)
  line L56 (-11.6619, -19.2129) -> (-4.6477, -16.2732)
  line L57 (-4.6477, -16.2732) -> (-3.0669, -8.2665)
  line L58 (-3.0669, -8.2665) -> (-0.0042, -8.2665)
  line L59 (11.3927, -55.7681) -> (12.0953, -55.4053)
  line L60 (12.0953, -55.4053) -> (18.2688, -59.6322)
  line L61 (18.2688, -59.6322) -> (22.3017, -55.5464)
  line L62 (22.3017, -55.5464) -> (18.0055, -49.2252)
  line L63 (18.0055, -49.2252) -> (21.1726, -41.4452)
  line L64 (21.1726, -41.4452) -> (28.7782, -40.0379)
  line L65 (28.7782, -40.0379) -> (28.7782, -34.318)
  line L66 (28.7782, -34.318) -> (21.1167, -32.8503)
  line L67 (21.1167, -32.8503) -> (17.8651, -25.3271)
  line L68 (17.8651, -25.3271) -> (22.3704, -18.7471)
  line L69 (22.3704, -18.7471) -> (18.2796, -14.7094)
  line L70 (18.2796, -14.7094) -> (11.6534, -19.2129)
  line L71 (11.6534, -19.2129) -> (4.6393, -16.2732)
  line L72 (4.6393, -16.2732) -> (3.0584, -8.2665)
  line L73 (3.0584, -8.2665) -> (-0.0042, -8.2665)
  line L74 (11.3927, -55.7681) -> (7.849, -57.5981)
  line L75 (-7.8574, -57.5981) -> (-7.986, -57.5317)
  line L76 (-3.1992, -45.3352) -> (-3.7536, -46.7702)
  line L77 (3.6756, -46.7973) -> (3.1212, -45.3624)
  line L78 (-9.2352, -56.8866) -> (-4.8785, -46.2449)
  line L79 (9.2267, -56.8866) -> (4.8701, -46.2449)
  point P0 (0, 0)
  point P1 (-18.614, -47.7512)
  point P2 (-20.6405, -42.7731)
  point P3 (-20.6078, -31.6532)
  point P4 (-18.2155, -26.1182)
  point P5 (-10.8284, -18.8636)
  point P6 (-5.541, -16.6475)
  point P7 (5.5325, -16.6475)
  point P8 (10.82, -18.8636)
  point P9 (18.207, -26.1182)
  point P10 (20.5993, -31.6532)
  point P11 (20.6321, -42.7731)
  point P12 (18.6055, -47.7512)
  point P13 (3.6756, -46.7973)
  point P14 (3.6756, -46.7973)
  point P15 (4.8701, -46.2449)
  point P16 (9.2267, -56.8866)
  dimension "d101" = 5.8166
  constraints: 150 end point, 35 symmetric about line, 8 perpendicular, 8 point on circle, 7 point on line, 3 centre point, 3 line through centre, 1 horizontal, 1 parallel, 1 vertical, 17 other
  measures "d101" distance between parallel lines of L4 L3
extrude "Extrusion15" add sketch "Sketch16" along normal blind 0.635 contours A0 L76 A1 L77 | A0 L5 A1 L76 | A1 L6 A2 L78 | A1 L79 A2 L25 | A2 L79 L74 L41 | L23 L43 L78 A2 | L74 L59 L60 L61 L62 L63 A2 L64 L65 L66 L67 L68 L69 L70 L71 L72 L73 L24 L26 L27 L28 L29 L30 L31 L32 L42 L33 L34 L35 L36 L37 L38 L39 L40 L41 | L23 L22 L21 L20 L19 L18 L17 L16 L15 L14 L13 L12 L11 L10 L9 L8 L7 L24 L58 L57 L56 A2 L55 L54 L53 L52 L51 L50 L49 L48 L47 L46 L45 L44 L43 | A2 L48 | L63 A2 | A2 L52 | L67 A2 | A2 L56 | L71 A2 bodies 3
extrude "Extrusion16" add sketch "Sketch16" along normal blind 1.27 contours L78 A2 L48 L52 L56 L71 L67 L63 L79 A1 | L78 L43 L44 L45 L46 L47 L48 A2 | A2 L63 L62 L61 L60 L59 L74 L79 | L48 L49 L50 L51 L52 A2 | A2 L67 L66 L65 L64 L63 | L52 L53 L54 L55 L56 A2 | A2 L71 L70 L69 L68 L67 | L56 L57 L58 L24 A2 | L24 L73 L72 L71 A2 bodies 3
sketch "Sketch17" plane through (0, 84.455, 0) normal (0, 1, 0) x (1, 0, 0)
  line L0 (-38.1, -61.8129) -> (-38.1, 61.8129) projected
  line L1 (-38.1, 0) -> (38.1, 0)
  line L2 (38.1, 0) -> (38.1, 73.025)
  line L3 (38.1, 73.025) -> (-38.1, 73.025)
  line L4 (-38.1, 73.025) -> (-38.1, 0)
  line L5 (-20.0063, 61.5126) -> (19.9937, 61.5126)
  line L6 (24.9937, 56.5125) -> (24.9937, 16.5126)
  line L7 (19.9937, 11.5126) -> (-20.0063, 11.5126)
  line L8 (-25.0063, 16.5126) -> (-25.0063, 56.5125)
  line L9 (-25.0063, 61.5126) -> (-19.5063, 61.5126)
  line L10 (-19.5063, 58.0626) -> (-19.5063, 56.0126)
  line L11 (-19.5063, 56.0126) -> (-21.5563, 56.0126)
  line L12 (-25.0063, 56.0126) -> (-25.0063, 61.5126)
  circle A0 centre (-19.5063, 56.0126) radius 2.05
  line L13 (-0.0063, 61.5126) -> (-0.0063, 59.165)
  line L14 (-25.0063, 36.5126) -> (-20.8648, 36.5126)
  circle A1 centre (19.4937, 56.0126) radius 2.05
  circle A2 centre (-19.5063, 17.0126) radius 2.05
  circle A3 centre (19.4937, 17.0126) radius 2.05
  arc A4 (-20.0063, 61.5126) -> (-25.0063, 56.5125) centre (-20.0063, 56.5125) ccw
  arc A5 (24.9937, 56.5125) -> (19.9937, 61.5126) centre (19.9937, 56.5125) ccw
  arc A6 (19.9937, 11.5126) -> (24.9937, 16.5126) centre (19.9937, 16.5126) ccw
  arc A7 (-25.0063, 16.5126) -> (-20.0063, 11.5126) centre (-20.0063, 16.5126) ccw
  line L15 (19.9937, 62.7829) -> (-20.0063, 62.7829)
  arc A8 (-20.0063, 62.7829) -> (-26.2766, 56.5125) centre (-20.0063, 56.5125) ccw
  line L16 (-26.2766, 56.5125) -> (-26.2766, 16.5126)
  arc A9 (-26.2766, 16.5126) -> (-20.0063, 10.2422) centre (-20.0063, 16.5126) ccw
  line L17 (-20.0063, 10.2422) -> (19.9937, 10.2422)
  arc A10 (19.9937, 10.2422) -> (26.264, 16.5126) centre (19.9937, 16.5126) ccw
  line L18 (26.264, 16.5126) -> (26.264, 56.5125)
  arc A11 (26.264, 56.5125) -> (19.9937, 62.7829) centre (19.9937, 56.5125) ccw
  point P0 (0, 0)
  point P1 (24.9937, 11.5126)
  point P2 (24.9937, 61.5126)
  point P3 (-25.0063, 11.5126)
  dimension "d118" = 50
  dimension "d119" = 50
  dimension "d120" = 13.0937
  dimension "d121" = 11.5125
  dimension "d123" = 5.5
  dimension "d124" = 5.5
  dimension "d125" = 4.1
  dimension "d128" = 5
  constraints: 36 end point, 18 point on circle, 12 centre point, 8 parallel, 8 point on line, 8 tangent, 4 horizontal, 4 perpendicular, 3 equal radius, 3 midpoint, 3 symmetric about line, 1 coincident, 1 vertical, 10 other
  measures "d118" distance of point (24.994, 11.513) point (-25.006, 11.513)
  measures "d119" distance of point (24.994, 61.513) point (24.994, 11.513)
  measures "d120" distance between parallel lines of L0 L8
  measures "d121" distance between parallel lines of L1 L7
  measures "d123" distance of L10.end L12.start
  measures "d124" distance of L9.end L10.end
  measures "d125" diameter of A0
  measures "d128" radius of A4
extrude "Extrusion17" add sketch "Sketch17" along normal up to surface (0.635 mm away) contours L9 A8 L15 A11 L18 A10 L17 A9 L16 L12 L8 A7 L7 A6 L6 A5 L5 | A4 L12 A8 L9 | L5 A5 L6 A6 L7 A7 L8 A4 bodies 3
sketch "Sketch18" plane through (-20.0063, 85.09, -10.2422) normal (0, 1, 0) x (1, 0, 0)
  arc A0 (0, 52.5406) -> (-6.2703, 46.2703) centre (0, 46.2703) ccw projected
  line L0 (-6.2703, 6.2703) -> (-6.2703, 46.2703) projected
  arc A1 (-6.2703, 6.2703) -> (0, 0) centre (0, 6.2703) ccw projected
  line L1 (40, 0) -> (0, 0) projected
  arc A2 (40, 0) -> (46.2703, 6.2703) centre (40, 6.2703) ccw projected
  line L2 (46.2703, 46.2703) -> (46.2703, 6.2703) projected
  arc A3 (46.2703, 46.2703) -> (40, 52.5406) centre (40, 46.2703) ccw projected
  line L3 (0, 52.5406) -> (40, 52.5406) projected
  circle A4 centre (39.5, 45.7703) radius 2.05 projected
  circle A5 centre (0.5, 6.7703) radius 2.05 projected
  circle A6 centre (39.5, 6.7703) radius 2.05 projected
  circle A7 centre (0.5, 45.7703) radius 2.05 projected
  circle A8 centre (20, 26.2703) radius 6.223
  circle A9 centre (20, 26.2703) radius 11.303
  circle A10 centre (20, 26.2703) radius 12.573
  circle A11 centre (20, 26.2703) radius 17.653
  circle A12 centre (20, 26.2703) radius 18.923
  circle A13 centre (20, 26.2703) radius 24.003
  line L4 (-6.2703, 52.5406) -> (46.2703, 52.5406)
  line L5 (46.2703, 52.5406) -> (46.2703, 0)
  line L6 (46.2703, 0) -> (-6.2703, 0)
  line L7 (-6.2703, 0) -> (-6.2703, 52.5406)
  line L8 (-6.2703, 52.5406) -> (-4.149, 52.5406)
  line L9 (-6.2703, 52.5406) -> (-6.2703, 50.4193)
  line L10 (-6.2703, 50.4193) -> (-4.149, 52.5406)
  line L11 (46.2703, 52.5406) -> (45.4995, 51.7698)
  line L12 (46.2703, 0) -> (46.2703, 2.1213)
  line L13 (46.2703, 0) -> (44.149, 0)
  line L14 (44.149, 0) -> (46.2703, 2.1213)
  line L15 (-4.149, 52.5406) -> (4.1212, 44.2705)
  line L16 (7.7222, 40.6695) -> (4.1212, 44.2705)
  line L17 (7.7222, 40.6695) -> (8.6232, 39.7684)
  line L18 (8.6232, 39.7684) -> (12.2337, 36.1579)
  line L19 (12.2337, 36.1579) -> (13.1389, 35.2527)
  line L20 (13.1389, 35.2527) -> (16.7901, 31.6016)
  line L21 (16.7901, 31.6016) -> (25.3312, 23.0604)
  line L22 (25.3312, 23.0604) -> (28.9824, 19.4092)
  line L23 (28.9824, 19.4092) -> (29.8876, 18.504)
  line L24 (33.4981, 14.8936) -> (29.8876, 18.504)
  line L25 (33.4981, 14.8936) -> (34.3991, 13.9925)
  line L26 (34.3991, 13.9925) -> (38.0002, 10.3915)
  line L27 (38.0002, 10.3915) -> (46.2703, 2.1213)
  line L28 (20, 26.2703) -> (18.9393, 27.331)
  line L29 (-6.2703, 50.4193) -> (1.9998, 42.1492)
  line L30 (5.6009, 38.5481) -> (1.9998, 42.1492)
  line L31 (5.6009, 38.5481) -> (6.5019, 37.6471)
  line L32 (6.5019, 37.6471) -> (10.1124, 34.0366)
  line L33 (10.1124, 34.0366) -> (11.0176, 33.1314)
  line L34 (11.0176, 33.1314) -> (14.6688, 29.4802)
  line L35 (14.6688, 29.4802) -> (23.2099, 20.9391)
  line L36 (23.2099, 20.9391) -> (26.8611, 17.2879)
  line L37 (26.8611, 17.2879) -> (27.7663, 16.3827)
  line L38 (31.3768, 12.7722) -> (27.7663, 16.3827)
  line L39 (31.3768, 12.7722) -> (32.2778, 11.8712)
  line L40 (32.2778, 11.8712) -> (35.8788, 8.2701)
  line L41 (35.8788, 8.2701) -> (44.149, 0)
  line L42 (20, 26.2703) -> (20, 25.9187)
  line L43 (44.149, 52.5406) -> (35.8788, 44.2705)
  line L44 (32.2778, 40.6695) -> (35.8788, 44.2705)
  line L45 (32.2778, 40.6695) -> (31.3768, 39.7684)
  line L46 (31.3768, 39.7684) -> (27.7663, 36.1579)
  line L47 (27.7663, 36.1579) -> (26.8611, 35.2527)
  line L48 (26.8611, 35.2527) -> (23.2099, 31.6016)
  line L49 (23.2099, 31.6016) -> (14.6688, 23.0604)
  line L50 (14.6688, 23.0604) -> (11.0176, 19.4092)
  line L51 (11.0176, 19.4092) -> (10.1124, 18.504)
  line L52 (6.5019, 14.8936) -> (10.1124, 18.504)
  line L53 (6.5019, 14.8936) -> (5.6009, 13.9925)
  line L54 (5.6009, 13.9925) -> (1.9998, 10.3915)
  line L55 (1.9998, 10.3915) -> (-6.2703, 2.1213)
  line L56 (25.3312, 29.4802) -> (16.7901, 20.9391)
  line L57 (28.9824, 33.1314) -> (25.3312, 29.4802)
  line L58 (33.4981, 37.6471) -> (29.8876, 34.0366)
  line L59 (29.8876, 34.0366) -> (28.9824, 33.1314)
  line L60 (34.3991, 38.5481) -> (33.4981, 37.6471)
  line L61 (34.3991, 38.5481) -> (38.0002, 42.1492)
  line L62 (46.2703, 50.4193) -> (38.0002, 42.1492)
  line L63 (7.7222, 11.8712) -> (4.1212, 8.2701)
  line L64 (8.6232, 12.7722) -> (7.7222, 11.8712)
  line L65 (8.6232, 12.7722) -> (12.2337, 16.3827)
  line L66 (13.1389, 17.2879) -> (12.2337, 16.3827)
  line L67 (16.7901, 20.9391) -> (13.1389, 17.2879)
  line L68 (4.1212, 8.2701) -> (-4.149, 0)
  point P0 (20.0063, -10.2422)
  point P1 (31.3768, 39.7684)
  point P2 (23.2099, 31.6016)
  point P3 (6.5019, 14.8936)
  point P4 (13.1389, 17.2879)
  point P5 (26.8611, 17.2879)
  point P6 (31.3768, 12.7722)
  point P7 (27.7663, 16.3827)
  point P8 (7.7222, 11.8712)
  point P9 (4.1212, 8.2701)
  point P10 (35.8788, 8.2701)
  point P11 (32.2778, 11.8712)
  point P12 (38.0002, 42.1492)
  point P13 (34.3991, 38.5481)
  point P14 (5.6009, 13.9925)
  dimension "d131" = 12.446
  dimension "d132" = 5.08
  dimension "d133" = 1.27
  dimension "d134" = 5.08
  dimension "d135" = 1.27
  dimension "d136" = 5.08
  dimension "d140" = 2.1213
  dimension "d141" = 2.1213
  constraints: 130 end point, 47 point on line, 42 symmetric about line, 12 point on circle, 6 centre point, 3 parallel, 2 collinear, 2 perpendicular, 1 horizontal, 1 vertical
  measures "d131" diameter of A8
  measures "d132" radial gap between concentric circles of A8 A9
  measures "d133" radial gap between concentric circles of A9 A10
  measures "d134" radial gap between concentric circles of A10 A11
  measures "d135" radial gap between concentric circles of A11 A12
  measures "d136" radial gap between concentric circles of A12 A13
  measures "d140" distance of L4.start L8.end
  measures "d141" distance of L4.start L9.end
extrude "Extrusion19" cut sketch "Sketch18" against normal blind 25.4 contours L15 A7 L29 | A7 L15 | L29 A7 | L43 A4 | A4 L62 L43 | A4 L62 | L55 A5 L68 | A5 L55 | L68 A5 | L27 A6 | A6 L41 L27 | A6 L41 bodies 3
sketch "Sketch19" plane through (-20.0063, 85.09, -10.2422) normal (0, 1, 0) x (1, 0, 0)
  arc A0 (0, 52.5406) -> (-6.2703, 46.2703) centre (0, 46.2703) ccw projected
  line L0 (-6.2703, 6.2703) -> (-6.2703, 46.2703) projected
  arc A1 (-6.2703, 6.2703) -> (0, 0) centre (0, 6.2703) ccw projected
  line L1 (40, 0) -> (0, 0) projected
  arc A2 (40, 0) -> (46.2703, 6.2703) centre (40, 6.2703) ccw projected
  line L2 (46.2703, 46.2703) -> (46.2703, 6.2703) projected
  arc A3 (46.2703, 46.2703) -> (40, 52.5406) centre (40, 46.2703) ccw projected
  line L3 (0, 52.5406) -> (40, 52.5406) projected
  circle A4 centre (39.5, 45.7703) radius 2.05 projected
  circle A5 centre (0.5, 6.7703) radius 2.05 projected
  circle A6 centre (39.5, 6.7703) radius 2.05 projected
  circle A7 centre (0.5, 45.7703) radius 2.05 projected
  point P0 (20.0063, -10.2422)
extrude "Extrusion20" add sketch "Sketch19" along normal blind 0.635 bodies 3